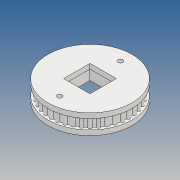
# Autodesk Inventor part: polea pequeña
Saved by Autodesk Inventor 2017 (Build 210142000, 142)
## iProperties
Part Number: polea pequeña
Material: Genérico
Document SubType Name: Modeling
Designer: FABLAB
Density: 1 g/cm^3
Appearance: Blanco
Description: Acrílico corte laser CNC
Author: FABLAB
Autodesk Inventor part; units mm, degrees
ref_plane "YZ Plane" through (0, 0, 0) normal (1, 0, 0) x (0, 1, 0)
ref_plane "XZ Plane" through (0, 0, 0) normal (0, 1, 0) x (-1, 0, 0)
ref_plane "XY Plane" through (0, 0, 0) normal (0, 0, 1) x (1, 0, 0)
sketch "Boceto1" plane through (0, 0, 0) normal (0, 0, 1) x (1, 0, 0)
  line L0 (8, -8) -> (-8, -8) projected
  line L1 (-8, -8) -> (-8, 8) projected
  line L2 (-8, 8) -> (8, 8) projected
  line L3 (8, 8) -> (8, -8) projected
  circle A0 centre (0, 0) radius 15 construction
  circle A1 centre (0, 0) radius 23.45
  circle A2 centre (0, 0) radius 18.45 construction
  circle A3 centre (0, 18.45) radius 1.5
  circle A4 centre (0, -18.45) radius 1.5
  circle A5 centre (0, 23.45) radius 1
  circle A6 centre (-3.6684, 23.1613) radius 1
  circle A7 centre (-7.2464, 22.3023) radius 1
  circle A8 centre (-10.6461, 20.8941) radius 1
  circle A9 centre (-13.7836, 18.9714) radius 1
  circle A10 centre (-16.5817, 16.5817) radius 1
  circle A11 centre (-18.9714, 13.7836) radius 1
  circle A12 centre (-20.8941, 10.6461) radius 1
  circle A13 centre (-22.3023, 7.2464) radius 1
  circle A14 centre (-23.1613, 3.6684) radius 1
  circle A15 centre (-23.45, 0) radius 1
  circle A16 centre (-23.1613, -3.6684) radius 1
  circle A17 centre (-22.3023, -7.2464) radius 1
  circle A18 centre (-20.8941, -10.6461) radius 1
  circle A19 centre (-18.9714, -13.7836) radius 1
  circle A20 centre (-16.5817, -16.5817) radius 1
  circle A21 centre (-13.7836, -18.9714) radius 1
  circle A22 centre (-10.6461, -20.8941) radius 1
  circle A23 centre (-7.2464, -22.3023) radius 1
  circle A24 centre (-3.6684, -23.1613) radius 1
  circle A25 centre (0, -23.45) radius 1
  circle A26 centre (3.6684, -23.1613) radius 1
  circle A27 centre (7.2464, -22.3023) radius 1
  circle A28 centre (10.6461, -20.8941) radius 1
  circle A29 centre (13.7836, -18.9714) radius 1
  circle A30 centre (16.5817, -16.5817) radius 1
  circle A31 centre (18.9714, -13.7836) radius 1
  circle A32 centre (20.8941, -10.6461) radius 1
  circle A33 centre (22.3023, -7.2464) radius 1
  circle A34 centre (23.1613, -3.6684) radius 1
  circle A35 centre (23.45, 0) radius 1
  circle A36 centre (23.1613, 3.6684) radius 1
  circle A37 centre (22.3023, 7.2464) radius 1
  circle A38 centre (20.8941, 10.6461) radius 1
  circle A39 centre (18.9714, 13.7836) radius 1
  circle A40 centre (16.5817, 16.5817) radius 1
  circle A41 centre (13.7836, 18.9714) radius 1
  circle A42 centre (10.6461, 20.8941) radius 1
  circle A43 centre (7.2464, 22.3023) radius 1
  circle A44 centre (3.6684, 23.1613) radius 1
  circle A45 centre (0, 0) radius 24.45 construction
  dimension "d0" = 46.9
  dimension "d4" = 5
  dimension "d3" = 3
  dimension "d7" = 360
  dimension "d16" = 2
  dimension "d19" = 360
  dimension "d24" = 48.9
  constraints: 43 centre point, 4 vertical alignment, 3 coincident, 1 tangent, 90 other
  measures "d3" diameter of A3
  measures "d16" diameter of A5
  measures "d24" diameter of A45
extrude "Extrusión1" add sketch "Boceto1" along normal blind 6
sketch "Boceto2" plane through (0, 0, 0) normal (0, 0, -1) x (-1, 0, 0)
  circle A0 centre (0, 0) radius 25.5
  circle A1 centre (0, 0) radius 15.5
  circle A2 centre (0, 18.45) radius 1.5 projected
  circle A3 centre (0, -18.45) radius 1.5 projected
  dimension "d9" = 31
  dimension "d21" = 51
  constraints: 3 coincident, 2 centre point
  measures "d9" diameter of A1
  measures "d21" diameter of A0
extrude "Extrusión2" add sketch "Boceto2" along normal blind 3 separate body
sketch "Boceto3" plane through (0, 0, 6) normal (0, 0, 1) x (1, 0, 0)
  circle A0 centre (0, 0) radius 25.5 projected
  circle A1 centre (0, 18.45) radius 1.5 projected
  circle A2 centre (0, -18.45) radius 1.5 projected
  line L0 (8, 8) -> (-8, 8) projected
  line L1 (8, -8) -> (8, 8) projected
  line L2 (-8, -8) -> (8, -8) projected
  line L3 (-8, 8) -> (-8, -8) projected
extrude "Extrusión3" add sketch "Boceto3" along normal blind 3 separate body
